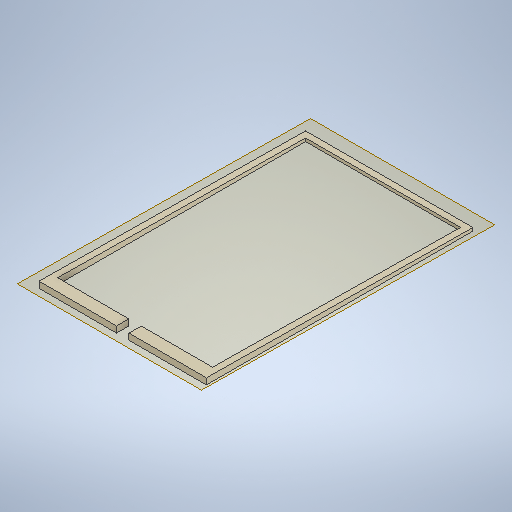
# Autodesk Inventor part: wing0.3.1_conductive
Saved by Autodesk Inventor 2025 (Build 290162000, 162)
## iProperties
Created: 2026-06-11
Part Number: wing0.3.1_conductive
Material: Generic
Document SubType Name: Modeling
Designer: DSTJOHN
Density: 1 g/cm^3
Appearance: Default
Author: DSTJOHN
Autodesk Inventor part; units mm, degrees
ref_plane "YZ Plane" through (0, 0, 0) normal (1, 0, 0) x (0, 1, 0)
ref_plane "XZ Plane" through (0, 0, 0) normal (0, 1, 0) x (-1, 0, 0)
ref_plane "XY Plane" through (0, 0, 0) normal (0, 0, 1) x (1, 0, 0)
sketch "Sketch1" plane through (0, 0, 0) normal (0, 1, 0) x (-1, 0, 0)
  line L0 (-54, 0) -> (-54, -86)
  line L1 (-54, -86) -> (0, -86)
  line L2 (0, -86) -> (0, 0)
  line L3 (0, 0) -> (-2, 0) construction
  line L4 (-2, 0) -> (-2, -4) construction
  line L5 (0, -86) -> (0, -84) construction
  line L6 (-52, -4) -> (-52, -84)
  line L7 (-52, -84) -> (-2, -84)
  line L8 (-2, -84) -> (-2, -4)
  line L9 (-25, 0) -> (-25, -4)
  line L10 (-29, 0) -> (-29, -4)
  line L11 (-2, -4) -> (-25, -4)
  line L12 (-29, -4) -> (-52, -4)
  line L13 (0, 0) -> (-25, 0)
  line L14 (-29, 0) -> (-54, 0)
  point P0 (-25, -2)
  dimension "d1" = 54
  dimension "d2" = 86
  dimension "d3" = 2
  dimension "d4" = 4
  dimension "d5" = 2
  dimension "d6" = 50
  dimension "d7" = 25
  dimension "d8" = 29
  constraints: 30 end point, 8 perpendicular, 7 parallel, 4 horizontal, 2 point on line, 1 midpoint
  measures "d1" distance of L1.end L0.end
  measures "d2" distance of L0.end L0.start
  measures "d3" distance of L2.end L3.end
  measures "d4" distance of L3.end L4.end
  measures "d5" distance of L1.end L5.end
  measures "d6" distance of L7.end L6.end
  measures "d7" distance from line of point (-25, -2) L2
  measures "d8" distance between parallel lines of L10 L2
extrude "Extrusion1" add sketch "Sketch1" along normal blind 2
ref_plane "Work Plane1" through (0, 2, 0) normal (0, 0.9999, -0.0118) x (1, 0, 0)
sketch "Sketch2" plane through (0, 2, 0) normal (0, 0.9999, -0.0118) x (1, 0, 0)
  line L0 (-35.8906, -24.3728) -> (94.8707, -24.3728)
  line L1 (94.8707, -24.3728) -> (94.8707, 112.0739)
  line L2 (94.8707, 112.0739) -> (-35.8906, 112.0739)
  line L3 (-35.8906, 112.0739) -> (-35.8906, -24.3728)
  point P0 (0, 0.0236)
  constraints: 8 end point, 2 parallel, 1 horizontal, 1 perpendicular
extrude "Extrusion2" cut sketch "Sketch2" along normal blind 8.25
body "Solid1"
